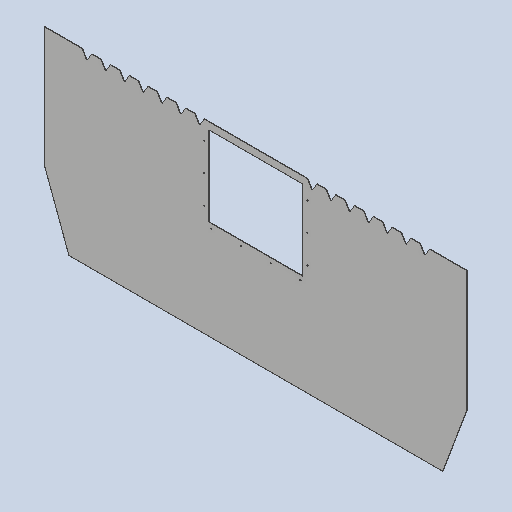
# Autodesk Inventor part: MSC 072 ridge 2
Saved by Autodesk Inventor 2025 (Build 290162010, 162A)
## iProperties
Created: 2024-06-08
Part Number: MSC 072 ridge 2
Material: Generic
Document SubType Name: Sheet Metal
Designer: admin
Density: 1 g/cm^3
Sheet Metal Rule: Default
Appearance: Default
Stock Number: МОО 072 гребень 2
Author: admin
Autodesk Inventor part; units mm, degrees
ref_plane "YZ Plane" through (0, 0, 0) normal (1, 0, 0) x (0, 1, 0)
ref_plane "XZ Plane" through (0, 0, 0) normal (0, 1, 0) x (-1, 0, 0)
ref_plane "XY Plane" through (0, 0, 0) normal (0, 0, 1) x (1, 0, 0)
sketch "Sketch1" plane through (0, 0, 0) normal (0, 1, 0) x (-1, 0, 0)
  line L0 (-900, 0) -> (-900, -513)
  line L1 (-900, -513) -> (-796.3397, -791.8723)
  line L2 (0, -791.8723) -> (0, 0)
  line L3 (0, 0) -> (-900, 0)
  line L4 (0, -370) -> (-200, -370)
  line L5 (-200, -370) -> (-200, 0)
  line L6 (-796.3397, -791.8723) -> (0, -791.8723)
  line L7 (-200, -30) -> (0, -30)
  dimension "d0" = 513
  dimension "d2" = 791.872
  dimension "d6" = 200
  dimension "d19" = 370
  dimension "d23" = 900
  dimension "d43" = 30
  measures "d0" distance of L0.start L0.end
  measures "d2" distance of L2.start L2.end
  measures "d6" distance between parallel lines of L2 L5
  measures "d19" distance of L4.end L5.end
  measures "d23" distance between parallel lines of L0 L2
  measures "d43" distance between parallel lines of L7 L3
extrude "Plate1" add sketch "Sketch1" along normal blind 2 contours L3 L5 L4 L2 L6 L1 L0 | L3 L2 L7 L5
sketch "Sketch5" plane through (0, 2, 0) normal (0, 1, 0) x (1, 0, 0)
  line L0 (900, 0) -> (0, 0) projected
  line L1 (900, 513) -> (900, 0) projected
  line L2 (796.3397, 791.8723) -> (900, 513) projected
  line L3 (0, 791.8723) -> (796.3397, 791.8723) projected
  line L4 (0, 370) -> (0, 791.8723) projected
  line L5 (200, 370) -> (0, 370) projected
  line L6 (200, 30) -> (200, 370) projected
  line L7 (0, 0) -> (900, 0) projected
  line L8 (220, 0) -> (237.5, 30)
  line L9 (237.5, 30) -> (242.5, 30)
  line L10 (242.5, 30) -> (260, 0)
  line L11 (0, 30) -> (200, 30) projected
  line L12 (0, 0) -> (0, 30) projected
  point P0 (260, 0)
  dimension "d34" = 30
  dimension "d35" = 5
  dimension "d36" = 40
  dimension "d44" = 20
  constraints: 6 end point, 2 point on line, 1 equal length, 1 parallel
  measures "d34" distance between parallel lines of L9 L0
  measures "d35" distance of L8.end L9.end
  measures "d36" distance of L8.start L10.end
  measures "d44" distance from line of L8.start L6
extrude "Extrusion1" cut sketch "Sketch5" against normal through all contours L0 L8 L9 L10
pattern_linear "Rectangular Pattern1" count 7 spacing 80 along (1, 0, 0) of "Extrusion1"
sketch "Sketch7" plane through (0, 2, 0) normal (0, 1, 0) x (1, 0, 0)
  line L0 (220, 80) -> (220, 320) construction
  line L1 (190, 390) -> (63.3333, 390) construction
  line L2 (200, 30) -> (200, 370) construction
  line L3 (200, 370) -> (0, 370) construction
  point P0 (0, 0)
  point P1 (220, 200)
  point P2 (200, 200)
  dimension "d45" = 20
  dimension "d46" = 240
  dimension "d47" = 10
  dimension "d48" = 20
  dimension "d49" = 190
  dimension "d50" = 126.6667
  constraints: 4 coincident, 4 end point, 2 midpoint, 1 horizontal, 1 horizontal alignment, 1 vertical
  measures "d45" distance between parallel lines of L0 L2
  measures "d46" distance of L0.start L0.end
  measures "d47" distance from line of point (190, 390) L2
  measures "d48" distance between parallel lines of L1 L3
  measures "d49" horizontal distance of L3.end point (190, 390)
  measures "d50" distance of point (190, 390) point (63.333, 390)
hole "Hole1" at (220, 2, -80) at (220, 2, -200) at (220, 2, -320) at (190, 2, -390) at (63.3333, 2, -390) direction (0, -1, 0) diameter 5.1 end through all
mirror "Mirror1" about plane through (0, 0, 0) normal (1, 0, 0) of "Plate1", "Extrusion1", "Rectangular Pattern1", "Hole1"
equation "\"d48\" = d45"
equation "\"d50\" = 0.666667 * d49"
equation "\"d56\" = Thickness"
equation "\"d3\" = Thickness"
equation "\"BendRadius\" = Thickness"
equation "\"BendReliefWidth\" = Thickness"
equation "\"BendReliefDepth\" = 0.5 * Thickness"
equation "\"CornerReliefSize\" = 4 * Thickness"
equation "\"MinimumRemnant\" = 2 * Thickness"
equation "\"TransitionRadius\" = BendRadius"
equation "\"JacobiRadiusSize\" = BendRadius"
equation "\"GapSize\" = Thickness"
equation "\"Thickness\" = 2"
body "Solid1"
